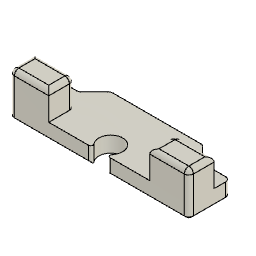
Handlebar Spacer (Autodesk Fusion 360 design; units mm, degrees)
Autodesk Fusion 360 part; units mm, degrees
sketch "Sketch1" plane through (0, 0, 0) normal (0, 0, 1) x (1, 0, 0)
  line L0 (19.5, 10) -> (-19.5, 10)
  line L1 (-19.5, 10) -> (-19.5, -10)
  line L2 (-19.5, -10) -> (19.5, -10)
  line L3 (19.5, -10) -> (19.5, 10)
  line L4 (19.5, 10) -> (-19.5, -10) construction
  line L5 (-19.5, 10) -> (19.5, -10) construction
  circle A0 centre (0, 0) radius 2.6
  dimension "d1" = 5.2
  dimension "d2" = 39
  dimension "d3" = 20
  constraint horizontal L0
  constraint perpendicular L0 L1
  constraint parallel L0 L2
  constraint parallel L1 L3
  constraint coincident L4 A0.centre
  constraint coincident L5 A0.centre
  constraint coincident A0.centre origin
  measures "d1" diameter of A0
  measures "d2" distance of L0.start L0.end
  measures "d3" distance of L0.start L2.end
extrude "Extrude1" add sketch "Sketch1" along normal blind 3.4
sketch "Sketch2" plane through (0, 0, 3.4) normal (0, 0, 1) x (-1, 0, 0)
  circle A0 centre (0, 0) radius 2.6
  line L0 (-19.5, 10) -> (-19.5, -10)
  line L1 (-19.5, -10) -> (19.5, -10)
  line L2 (19.5, -10) -> (19.5, 10)
  line L3 (19.5, 10) -> (-19.5, 10)
  line L4 (19.5, 3) -> (-19.5, 3)
  line L5 (19.5, -3) -> (-19.5, -3)
  line L6 (-19.5, 3) -> (19.5, -3) construction
  dimension "d7" = 6
  constraint coincident L2 L4.start
  constraint coincident L0 L4.end
  constraint perpendicular L0 L4
  constraint coincident L2 L5.start
  constraint coincident L0 L5.end
  constraint perpendicular L0 L5
  constraint coincident A0.centre L6
  measures "d7" distance of L4 L5
extrude "Extrude2" add sketch "Sketch2" along normal blind 6 contours L0 L2 L4 L5
extrude "Extrude5" cut 1 faces at (-6.5, -10, 2.2667) along direction (0, 1, 0) up to surface (7 mm away)
sketch "Sketch3" plane through (0, 0, 9.4) normal (0, 0, 1) x (-1, 0, 0)
  line L0 (19.5, 3) -> (-19.5, 3)
  line L1 (-19.5, 3) -> (-19.5, -3)
  line L2 (-19.5, -3) -> (19.5, -3)
  line L3 (19.5, -3) -> (19.5, 3)
  line L4 (11, -3) -> (11, 3)
  line L5 (-11, -3) -> (-11, 3)
  circle A0 centre (0, 0) radius 2.6
  dimension "d11" = 11
  dimension "d12" = 11
  constraint coincident L2 L4.start
  constraint coincident L0 L4.end
  constraint perpendicular L0 L4
  constraint coincident L2 L5.start
  constraint coincident L0 L5.end
  constraint perpendicular L0 L5
  measures "d11" distance of A0.centre L4
  measures "d12" distance of A0.centre L5
extrude "Extrude3" cut sketch "Sketch3" against normal up to surface (6 mm away) contours L0 L2 L4 L5
extrude "Extrude4" cut 1 faces at (-16.6667, -3, 4.2667) along direction (0, 1, 0) blind 0.5
sketch "Sketch4" plane through (0, 0, 3.4) normal (0, 0, 1) x (-1, 0, 0)
  line L0 (11, 2.5) -> (0.7141, 2.5)
  arc A0 (-0.7141, 2.5) -> (0.7141, 2.5) centre (0, 0) ccw
  line L1 (-0.7141, 2.5) -> (-11, 2.5)
  line L2 (-11, 2.5) -> (-11, -3)
  line L3 (-11, -3) -> (-19.5, -3)
  line L4 (-19.5, -3) -> (-19.5, -10)
  line L5 (-19.5, -10) -> (19.5, -10)
  line L6 (19.5, -10) -> (19.5, -3)
  line L7 (19.5, -3) -> (11, -3)
  line L8 (11, -3) -> (11, 2.5)
  line L9 (10, -10) -> (13.5, -6.5)
  line L10 (13.5, -6.5) -> (19.5, -6.5)
  line L11 (-10, -10) -> (-13.5, -6.5)
  line L12 (-13.5, -6.5) -> (-19.5, -6.5)
  dimension "d24" = 20
  dimension "d25" = 3.5
  dimension "d26" = 3.5
  dimension "d27" = 135
  dimension "d28" = 135
  constraint coincident L5 L9.start
  constraint coincident L6 L10.end
  constraint perpendicular L6 L10
  constraint coincident L5 L11.start
  constraint coincident L4 L12.end
  constraint perpendicular L4 L12
  constraint equal L10 L12
  measures "d24" distance of L9.start L11.start
  measures "d25" distance of L5.end L10.end
  measures "d26" distance of L4.end L12.end
  measures "d27" angle of L9 L10
  measures "d28" angle of L11 L12
extrude "Extrude6" cut sketch "Sketch4" against normal through all contours L5 L6 L9 L10 | L4 L5 L11 L12
fillet "Fillet2" radius 1 10 edges at (-19.5, -2.5, 4.7) (19.5, -2.5, 4.7) (11, 3, 6.4) (-11, 3, 6.4) (19.5, 6.5, 1.7) (-19.5, 6.5, 1.7) (-10, 10, 1.7) (10, 10, 1.7) (-13.5, 6.5, 1.7) (13.5, 6.5, 1.7)
fillet "Fillet1" radius 1 8 edges at (-15.25, -2.5, 9.4) (-19.5, 0.25, 9.4) (-11, 0.25, 9.4) (-15.25, 3, 9.4) (11, 0.25, 9.4) (15.25, -2.5, 9.4) (15.25, 3, 9.4) (19.5, 0.25, 9.4)
chamfer "Chamfer1" distance 0.5 angle 45 3 edges at (-19.5, 3.75, 0) (0, 10, 0) (19.5, 3.75, 0)
fillet "Fillet3" radius 0.5 2 edges at (-0.7141, -2.5, 1.95) (0.7141, -2.5, 1.95)
